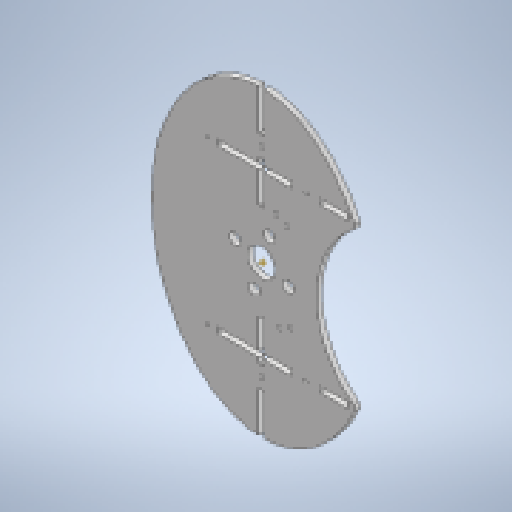
# Autodesk Inventor part: верхний эллипс туловища
Saved by Autodesk Inventor 2023 (Build 270158000, 158)
## iProperties
Created: 2024-11-21
Part Number: верхний эллипс туловища
Material: Типовые
Document SubType Name: Modeling
Designer: DELL
Density: 1 g/cm^3
Appearance: По умолчанию
Author: DELL
Autodesk Inventor part; units mm, degrees
ref_plane "YZ Plane" through (0, 0, 0) normal (1, 0, 0) x (0, 1, 0)
ref_plane "XZ Plane" through (0, 0, 0) normal (0, 1, 0) x (-1, 0, 0)
ref_plane "XY Plane" through (0, 0, 0) normal (0, 0, 1) x (1, 0, 0)
sketch "Эскиз1" plane through (0, 0, 0) normal (0, 0, 1) x (1, 0, 0)
  ellipse E0 centre (0, 0) end of major axis (2.1776, -109.9784) minor radius 80 (68.6548, 55.2754) -> (68.6548, -57.6949) ccw
  circle A0 centre (0, 0) radius 10
  line L0 (-129.1764, 146.988) -> (-129.1764, 142.988) construction
  line L1 (-149.1764, 146.9879) -> (-129.1764, 146.988) construction
  line L2 (-149.1764, 142.9879) -> (-149.1764, 146.9879) construction
  line L3 (-129.1764, 142.988) -> (-149.1764, 142.9879) construction
  line L4 (-169.9145, 146.9879) -> (-169.9145, 142.9879) construction
  line L5 (-189.9145, 146.9878) -> (-169.9145, 146.9879) construction
  line L6 (-189.9145, 142.9878) -> (-189.9145, 146.9878) construction
  line L7 (-169.9145, 142.9879) -> (-189.9145, 142.9878) construction
  arc A1 (68.6548, 55.2754) -> (68.6548, -57.6949) centre (110, -1.2098) ccw
  line L8 (68.6548, 55.2754) -> (68.6548, -57.6949) construction
  line L9 (0, 109.9808) -> (0, -109.9808) construction
  line L10 (-2, -110) -> (2, -110)
  line L11 (2, -110) -> (2, -80)
  line L12 (2, -80) -> (-2, -80)
  line L13 (-2, -80) -> (-2, -110)
  line L14 (2, -110) -> (-2, -80) construction
  point P0 (0, -95)
  point P1 (0, -110)
  point P2 (-2, -109.9112)
  point P3 (2, -109.9817)
  dimension "d0" = 110
  dimension "d1" = 80
  dimension "d4" = 20
  dimension "d19" = 70
  dimension "d21" = 110
  dimension "d24" = 4
  dimension "d25" = 30
  dimension "d26" = 110
  constraints: 30 end point, 4 coincident, 3 midpoint, 2 centre point, 2 parallel, 2 point on circle, 2 vertical, 1 horizontal, 1 perpendicular, 1 point on line, 6 other
  measures "d4" diameter of A0
  measures "d19" radius of A1
  measures "d21" horizontal distance of A0.centre A1.centre
  measures "d24" distance of L11.end L12.end
  measures "d25" distance of L10.end L11.end
  measures "d26" distance of point (0, 0) point (0, -110)
extrude "Выдавливание1" add sketch "Эскиз1" against normal blind 4 contours A1 E0 L11 L12 L13
fillet "Сопряжение1" radius 3 2 edges at (68.6548, 55.2754, -2) (68.6548, -57.6949, -2)
sketch "Эскиз5" plane through (0, 0, 0) normal (0, 0, 1) x (1, 0, 0)
  line L0 (-2, -110) -> (-2, -80)
  line L1 (-2, -80) -> (2, -80)
  line L2 (2, -80) -> (2, -110)
  line L3 (2, -110) -> (-2, -110)
  line L4 (-2, -34.6112) -> (2, -34.6112)
  line L5 (2, -64.6112) -> (-2, -64.6112)
  line L6 (-2, 65.3852) -> (2, 65.3852)
  line L7 (2, 35.3852) -> (-2, 35.3852)
  line L8 (-2, 80.7779) -> (-2, 110.7779)
  line L9 (-2, 110.7779) -> (2, 110.7779)
  line L10 (2, 110.7779) -> (2, 80.7779)
  line L11 (2, 80.7779) -> (-2, 80.7779)
  line L12 (-49.2252, -56.6111) -> (-46.452, -56.6111) construction
  line L13 (-46.452, -56.6111) -> (-46.452, -60.6111) construction
  line L14 (-46.452, -60.6111) -> (-49.2252, -60.6111) construction
  line L15 (-49.2252, -56.6111) -> (-49.2252, -60.6111) construction
  line L16 (-1.9986, -60.6111) -> (-31.9986, -60.6111)
  line L17 (-31.9986, -60.6111) -> (-31.9986, -56.6111)
  line L18 (-31.9986, -56.6111) -> (-1.9986, -56.6111)
  line L19 (2, -56.6111) -> (22.0269, -56.6111)
  line L20 (22.0269, -56.6111) -> (22.0269, -60.6111)
  line L21 (22.0269, -60.6111) -> (2, -60.6111)
  line L22 (42.765, -56.6111) -> (62.765, -56.6111)
  line L23 (62.765, -56.6111) -> (62.765, -60.6111)
  line L24 (62.765, -60.6111) -> (42.765, -60.6111)
  line L25 (42.765, -60.6111) -> (42.765, -56.6111)
  line L26 (-46.4535, 57.6183) -> (-49.2267, 57.6183) construction
  line L27 (-49.2267, 61.6183) -> (-49.2267, 57.6183) construction
  line L28 (-49.2267, 61.6183) -> (-46.4535, 61.6183) construction
  line L29 (-46.4535, 61.6183) -> (-46.4535, 57.6183) construction
  line L30 (-32.0001, 61.6183) -> (2, 61.6183)
  line L31 (-2.0001, 57.6186) -> (-2.0001, 57.6183)
  line L32 (2, 57.6183) -> (-32.0001, 57.6183)
  line L33 (-32.0001, 57.6183) -> (-32.0001, 61.6183)
  line L34 (62.7634, 61.6188) -> (62.7634, 57.6188)
  line L35 (42.7634, 61.6188) -> (62.7634, 61.6188)
  line L36 (62.7634, 57.6188) -> (42.7634, 57.6188)
  line L37 (42.7634, 57.6188) -> (42.7634, 61.6188)
  line L38 (22, 61.6187) -> (22, 57.6187)
  line L39 (22, 57.6187) -> (-2, 57.6186)
  line L40 (-2, 61.6186) -> (22, 61.6187)
  line L41 (-31.9986, -56.6111) -> (-46.452, -60.6111) construction
  circle A0 centre (-39.2253, -58.6111) radius 1.45
  line L42 (-2, -64.6112) -> (2, -80) construction
  circle A1 centre (0, -72.3056) radius 1.45
  line L43 (-46.4535, 57.6183) -> (-32.0001, 61.6183) construction
  circle A2 centre (-39.2268, 59.6183) radius 1.45
  line L44 (-2, 35.3852) -> (-2, 57.6186)
  line L45 (-2, 61.6183) -> (-2, 65.3852)
  line L46 (-2, -64.6112) -> (-2, -60.6111)
  line L47 (-2, -56.6111) -> (-2, -34.6112)
  line L48 (2, -34.6112) -> (2, -56.6111)
  line L49 (2, -60.6111) -> (2, -64.6112)
  line L50 (2, 65.3852) -> (2, 61.6186)
  line L51 (2, 57.6186) -> (2, 35.3852)
  line L52 (-2, 80.7779) -> (2, 65.3852) construction
  circle A3 centre (0, 73.0815) radius 1.45
  line L53 (2, 61.6186) -> (2, 57.6186)
  line L54 (-2, 57.6186) -> (-2, 61.6183)
  line L55 (2, -56.6111) -> (2, -60.6111)
  line L56 (-2, -60.6111) -> (-2, -56.6111)
  line L57 (42.7634, 61.6188) -> (22, 57.6187) construction
  circle A4 centre (32.3817, 59.6187) radius 1.45
  line L58 (42.765, -56.6111) -> (22.0269, -60.6111) construction
  circle A5 centre (32, -58.6874) radius 1.45
  point P0 (0, 0)
  point P1 (-2, 57.6183)
  dimension "d33" = 2.9
  dimension "d34" = 2.9
  dimension "d35" = 2.9
  dimension "d36" = 2.9
  dimension "d37" = 2.9
  dimension "d38" = 2.9
  constraints: 118 end point, 14 point on line, 6 centre point, 5 midpoint, 2 parallel, 2 vertical
  measures "d33" diameter of A0
  measures "d34" diameter of A1
  measures "d35" diameter of A2
  measures "d36" diameter of A3
  measures "d37" diameter of A4
  measures "d38" diameter of A5
extrude "Выдавливание3" cut sketch "Эскиз5" against normal blind 4
sketch "Эскиз7" plane through (0, 0, 0) normal (0, 0, 1) x (1, 0, 0)
  circle A0 centre (18.5161, 32.0336) radius 1.575 projected
  circle A1 centre (10.1981, 35.5668) radius 1.575 projected
  circle A2 centre (20.5676, -30.7567) radius 1.575 projected
  circle A3 centre (12.498, -34.8253) radius 1.575 projected
  circle A4 centre (19.2479, -5.433) radius 4 projected
  circle A5 centre (-5.433, -19.2479) radius 4 projected
  circle A6 centre (-19.2479, 5.433) radius 4 projected
  circle A7 centre (5.433, 19.2479) radius 4 projected
  point P0 (0, 0)
extrude "Выдавливание5" cut sketch "Эскиз7" against normal blind 10
